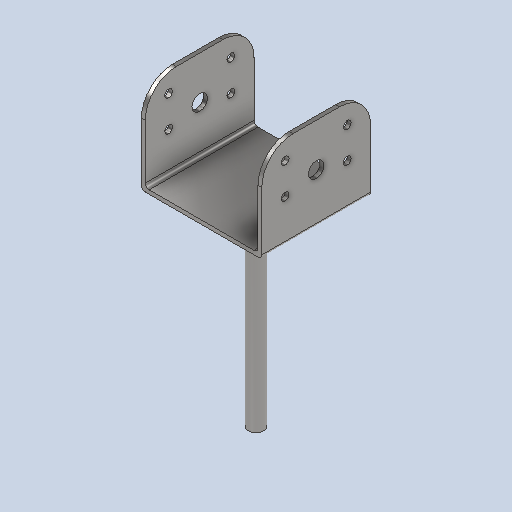
# Autodesk Inventor part: Saddle_Bracket
Saved by Autodesk Inventor 2025 (Build 290162010, 162A)
## iProperties
Created: 2024-09-15
Part Number: Saddle_Bracket
Material: Steel, Galvanized
Document SubType Name: Modeling
Designer: Tom
Density: 7.85 g/cm^3
Appearance: Galvanized
Author: Tom
Autodesk Inventor part; units mm, degrees
ref_plane "YZ Plane" through (0, 0, 0) normal (1, 0, 0) x (0, 1, 0)
ref_plane "XZ Plane" through (0, 0, 0) normal (0, 1, 0) x (-1, 0, 0)
ref_plane "XY Plane" through (0, 0, 0) normal (0, 0, 1) x (1, 0, 0)
sketch "Sketch1" plane through (0, 0, 0) normal (0, 1, 0) x (-1, 0, 0)
  line L0 (49.2125, 44.45) -> (-49.2125, 44.45)
  line L1 (-49.2125, 44.45) -> (-49.2125, -44.45)
  line L2 (-49.2125, -44.45) -> (49.2125, -44.45)
  line L3 (49.2125, -44.45) -> (49.2125, 44.45)
  line L4 (49.2125, 0) -> (-49.2125, 0)
  line L5 (0, -44.45) -> (0, 44.45)
  point P0 (0, 0)
  point P1 (0, 0)
  dimension "d0" = 98.425
  dimension "d1" = 88.9
  constraints: 12 end point, 5 midpoint, 2 parallel, 1 coincident, 1 horizontal, 1 perpendicular
  measures "d0" distance of L0.start L0.end
  measures "d1" distance of L2.end L0.start
extrude "Extrusion1" add sketch "Sketch1" along normal blind 3.175
sketch "Sketch2" plane through (0, 3.175, 0) normal (0, 1, 0) x (1, 0, 0)
  line L0 (49.2125, 44.45) -> (-49.2125, 44.45) projected
  line L1 (-49.2125, -44.45) -> (49.2125, -44.45) projected
  line L2 (49.2125, 44.45) -> (46.0375, 44.45)
  line L3 (46.0375, 44.45) -> (46.0375, -44.45)
  line L4 (46.0375, -44.45) -> (49.2125, -44.45)
  line L5 (49.2125, -44.45) -> (49.2125, 44.45)
  line L6 (-49.2125, 44.45) -> (-49.2125, -44.45) projected
  line L7 (-49.2125, 44.45) -> (-46.0375, 44.45)
  line L8 (-46.0375, 44.45) -> (-46.0375, -44.45)
  line L9 (-46.0375, -44.45) -> (-49.2125, -44.45)
  line L10 (-49.2125, -44.45) -> (-49.2125, 44.45)
  point P0 (0, 0)
  point P1 (-46.0375, -44.45)
  point P2 (-46.0375, 44.45)
  dimension "d4" = 3.175
  constraints: 16 end point, 4 parallel, 2 horizontal, 2 perpendicular, 2 point on line, 1 collinear
  measures "d4" distance between parallel lines of L8 L6
extrude "Extrusion2" add sketch "Sketch2" along normal blind 73.025 contours L5 L1 L3 L0 | L8 L1 L6 L0
fillet "Fillet1" radius 3.175 4 edges at (49.2125, 0, 0) (46.0375, 3.175, 0) (-49.2125, 0, 0) (-46.0375, 3.175, 0)
fillet "Fillet2" radius 25.4 4 edges at (47.625, 76.2, -44.45) (-47.625, 76.2, -44.45) (-47.625, 76.2, 44.45) (47.625, 76.2, 44.45)
sketch "Sketch3" plane through (49.2125, 3.175, 44.45) normal (1, 0, 0) x (0, 0, -1)
  circle A0 centre (69.85, 57.15) radius 3.175
  circle A1 centre (69.85, 31.75) radius 3.175
  line L0 (88.9, 0) -> (88.9, 47.625) projected
  line L1 (44.45, -3.175) -> (44.45, 73.025)
  line L2 (25.4, 73.025) -> (63.5, 73.025) projected
  circle A2 centre (19.05, 57.15) radius 3.175
  circle A3 centre (19.05, 31.75) radius 3.175
  circle A4 centre (44.45, 38.1) radius 6.35
  dimension "d10" = 6.35
  dimension "d11" = 19.05
  dimension "d12" = 15.875
  dimension "d13" = 25.4
  dimension "d14" = 19.05
  dimension "d15" = 12.7
  dimension "d16" = 6.35
  constraints: 5 centre point, 2 end point, 2 symmetric about line, 1 equal radius, 1 midpoint, 1 point on line, 2 other
  measures "d10" diameter of A0
  measures "d11" horizontal distance of L0.end A0.centre
  measures "d12" vertical distance of L2.end A0.centre
  measures "d13" distance of A0.centre A1.centre
  measures "d14" distance from line of L0 A1.centre
  measures "d15" diameter of A4
  measures "d16" vertical distance of A3.centre A4.centre
hole "Hole1" at (49.2125, 60.325, 25.4) at (49.2125, 60.325, -25.4) at (49.2125, 34.925, 25.4) at (49.2125, 34.925, -25.4) direction (-1, 0, 0) diameter 6.35 end through all
hole "Hole2" at (49.2125, 41.275, 0) direction (-1, 0, 0) diameter 12.7 end through all
sketch "Sketch4" plane through (0, 0, 0) normal (0, -1, 0) x (1, 0, 0)
  circle A0 centre (0, 0) radius 6.35
  dimension "d31" = 12.7
  constraints: 1 centre point, 1 coincident
  measures "d31" diameter of A0
extrude "Extrusion3" add sketch "Sketch4" along normal blind 165.1
body "Solid1"
